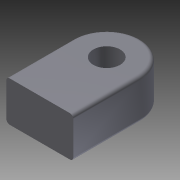
# Autodesk Inventor part: Lagar
Saved by Autodesk Inventor 2011 SP2 (Build 150309200, 309)
## iProperties
Created: 2023-03-20
Part Number: Lagar
Document SubType Name: Modeling
Designer: utilizator
Density: 1 g/cm^3
Author: utilizator
Autodesk Inventor part; units mm, degrees
ref_plane "YZ Plane" through (0, 0, 0) normal (1, 0, 0) x (0, 1, 0)
ref_plane "XZ Plane" through (0, 0, 0) normal (0, 1, 0) x (-1, 0, 0)
ref_plane "XY Plane" through (0, 0, 0) normal (0, 0, 1) x (1, 0, 0)
sketch "Sketch1" plane through (0, 0, 0) normal (0, 0, 1) x (1, 0, 0)
  line L0 (-28, 0) -> (28, 0) projected
  line L1 (0, -12) -> (0, 72) projected
  line L2 (-20, 60) -> (20, 60)
  line L3 (20, 60) -> (20, 0)
  line L4 (20, 0) -> (-20, 0)
  line L5 (-20, 0) -> (-20, 60)
  arc A0 (20, 40) -> (-20, 40) centre (0, 40) ccw
  line L6 (-20, 40) -> (20, 40) construction
  circle A1 centre (0, 40) radius 8
  point P0 (0, 0)
  point P1 (0, 60)
  point P2 (0, 0)
  dimension "d0" = 40
  dimension "d1" = 60
  dimension "d2" = 8
  constraints: 10 end point, 5 point on circle, 4 point on line, 3 coincident, 3 midpoint, 2 centre point, 2 parallel, 1 horizontal, 1 perpendicular, 1 vertical alignment
  measures "d0" distance of L3.end L4.end
  measures "d1" distance of L4.end L2.start
  measures "d2" radius of A1
extrude "Extrusion1" add sketch "Sketch1" along normal mid plane 24 contours L5 A0 L1 A1 L0 | L1 A1 A0 L3 L0
fillet "Fillet1" radius 2 8 edges at (20, 20, 12) (-14.1421, 54.1421, 12) (14.1421, 54.1421, 12) (-20, 20, 12) (20, 20, -12) (-14.1421, 54.1421, -12) (14.1421, 54.1421, -12) (-20, 20, -12)
body "Solid1"
